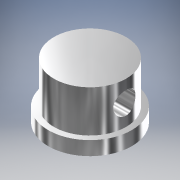
# Autodesk Inventor part: koncowka-wala
Saved by Autodesk Inventor 2017 (Build 210142000, 142)
## iProperties
Created: 2017-04-05
Part Number: koncowka-wala
Material: Aluminium 6061
Document SubType Name: Modeling
Designer: Dorota
Density: 2.7 g/cm^3
Appearance: Aluminium — płaski
Author: Dorota
Autodesk Inventor part; units mm, degrees
ref_plane "YZ Plane" through (0, 0, 0) normal (1, 0, 0) x (0, 1, 0)
ref_plane "XZ Plane" through (0, 0, 0) normal (0, 1, 0) x (-1, 0, 0)
ref_plane "XY Plane" through (0, 0, 0) normal (0, 0, 1) x (1, 0, 0)
sketch "Szkic1" plane through (0, 0, 0) normal (0, 0, 1) x (1, 0, 0)
  circle A0 centre (0, 0) radius 15
  dimension "d0" = 30
  constraints: 1 centre point, 1 coincident
  measures "d0" diameter of A0
extrude "Wyciągnięcie proste1" add sketch "Szkic1" along normal blind 5
sketch "Szkic2" plane through (0, 0, 5) normal (0, 0, 1) x (1, 0, 0)
  circle A0 centre (0, 0) radius 12.975
  dimension "d3" = 25.95
  constraints: 1 centre point, 1 coincident
  measures "d3" diameter of A0
extrude "Wyciągnięcie proste2" add sketch "Szkic2" along normal blind 15
sketch "Szkic3" plane through (0, 0, 0) normal (0, 1, 0) x (-1, 0, 0)
  circle A0 centre (0, 12.5) radius 1.5
  point P0 (0, 0)
  dimension "d6" = 3
  constraints: 1 centre point
  measures "d6" diameter of A0
extrude "Wyciągnięcie proste3" cut sketch "Szkic3" along normal blind 20
thread "Gwint1" size "M3x0.5" class "6H" standard "ANSI Metric M Profile" full length
sketch "Szkic4" plane through (0, 0, 0) normal (1, 0, 0) x (0, 1, 0)
  line L0 (0, 14) -> (0, 11) projected
  circle A0 centre (0, 12.5) radius 4
  point P0 (0, 0)
  dimension "d11" = 8
  constraints: 1 centre point, 1 midpoint
  measures "d11" diameter of A0
extrude "Wyciągnięcie proste4" cut sketch "Szkic4" along normal mid plane 35
